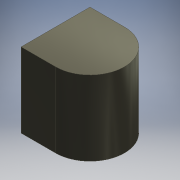
# Autodesk Inventor part: Belt Tensioner
Saved by Autodesk Inventor 2016 (Build 200138000, 138)
## iProperties
Created: 2017-02-03
Part Number: Belt Tensioner
Material: PC/ABS Plastic
Document SubType Name: Modeling
Designer: Scott
Density: 0.357273 g/cm^3
Appearance: Gunmetal
Author: Scott
## iProperties of the stored document Belt Tensioner_3DPrint.ipt
Created: 2017-04-15
Part Number: Belt Tensioner_3DPrint
Material: Generic
Document SubType Name: Modeling
Designer: Scott
Density: 1 g/cm^3
Appearance: Default
Author: Scott
Autodesk Inventor part; units mm, degrees
ref_plane "YZ Plane" through (0, 0, 0) normal (1, 0, 0) x (0, 1, 0)
ref_plane "XZ Plane" through (0, 0, 0) normal (0, 1, 0) x (-1, 0, 0)
ref_plane "XY Plane" through (0, 0, 0) normal (0, 0, 1) x (1, 0, 0)
sketch "Sketch1" plane through (0, 0, 0) normal (0, 0, 1) x (1, 0, 0)
  line L0 (0, 3) -> (3, 3)
  line L1 (6, 0) -> (6, 0)
  line L2 (3, -3) -> (0, -3)
  line L3 (0, -3) -> (0, 3)
  arc A0 (6, 0) -> (3, 3) centre (3, 0) ccw
  arc A1 (3, -3) -> (6, 0) centre (3, 0) ccw
  point P0 (0, 0)
  point P1 (0, 0)
  dimension "d0" = 3
  dimension "d1" = 6
  dimension "d2" = 6
  constraints: 8 end point, 4 point on circle, 4 tangent, 2 centre point, 2 parallel, 1 coincident, 1 concentric, 1 horizontal, 1 midpoint, 1 perpendicular
  measures "d0" radius of A0
  measures "d1" distance of L2.end L0.start
  measures "d2" distance from line of L1.start L3
extrude "Extrusion1" add sketch "Sketch1" along normal blind 6.5
sketch "Sketch2" plane through (0, -3, 0) normal (-1, 0, 0) x (0, 0, 1)
  line L0 (0, 6) -> (6.5, 6) projected
  line L1 (6.5, 6) -> (6.5, 0) projected
  line L2 (0, 0) -> (6.5, 0) projected
  line L3 (0, 0) -> (0, 6) projected
  line L4 (3.25, 6) -> (3.25, 0) construction
  line L5 (0, 3) -> (6.5, 3) construction
  point P0 (3.25, 3)
  constraints: 4 end point, 4 midpoint
hole "Hole1" at (0, 0, 3.25) direction (1, 0, 0) diameter 3.2 depth 2
body "Solid1"
